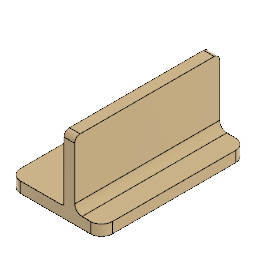
dc-dc-mount v2 (Autodesk Fusion 360 design; units mm, degrees)
Autodesk Fusion 360 part; units mm, degrees
sketch "Sketch1" plane through (0, 0, 0) normal (1, 0, 0) x (0, 1, 0)
  line L0 (0, 0) -> (40, 0)
  line L1 (40, 0) -> (40, 18)
  line L2 (40, 18) -> (0, 18)
  line L3 (0, 18) -> (0, 0)
  dimension "d1" = 40
  dimension "d2" = 18
  constraint horizontal L0
  constraint vertical L1
  constraint horizontal L2
  constraint vertical L3
  constraint coincident L0.start L3.end
  measures "d1" distance of L0.start L0.end
  measures "d2" distance of L0.start L2.end
extrude "Extrude1" add sketch "Sketch1" along normal blind 3
sketch "Sketch3" plane through (0, 0, 0) normal (0, 0, -1) x (1, 0, 0)
  line L0 (0, 0) -> (0, -40)
  line L1 (0, -40) -> (3, -40)
  line L2 (3, -40) -> (3, 0)
  line L3 (3, 0) -> (0, 0)
  line L4 (1.5, 0) -> (1.5, -40) construction
  line L5 (-15, -40) -> (10.4, -40)
  line L6 (10.4, -40) -> (10.4, 0)
  line L7 (10.4, 0) -> (-15, 0)
  line L8 (-15, 0) -> (-15, -40)
  dimension "d11" = 25.4
  dimension "d12" = 15
  constraint midpoint L3 L4.start
  constraint midpoint L1 L4.end
  constraint horizontal L5
  constraint vertical L6
  constraint horizontal L7
  constraint vertical L8
  constraint collinear L1 L5
  constraint collinear L3 L7
  measures "d11" distance of L5.start L5.end
  measures "d12" distance of L0 L8
extrude "Extrude3" add sketch "Sketch3" along normal blind 3
fillet "Fillet1" radius 3 4 edges at (-15, 40, -1.5) (-15, 0, -1.5) (10.4, 0, -1.5) (10.4, 40, -1.5)
fillet "Fillet2" radius 1.5 2 edges at (1.5, 40, 18) (1.5, 0, 18)
fillet "Fillet3" radius 2 1 edges at (3, 20, 0)
fillet "Fillet4" radius 0.5 1 edges at (0, 20, 0)
